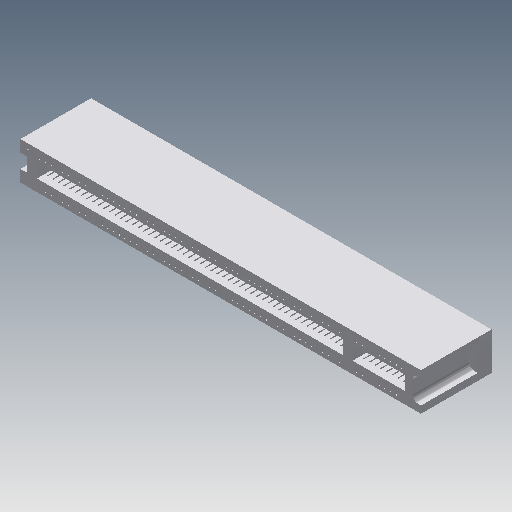
# Autodesk Inventor part: config - pci slot
Saved by Autodesk Inventor 2020 (Build 240152000, 152)
## iProperties
Created: 2005-12-05
Part Number: config - pci slot
Document SubType Name: Modeling
Designer: Simon.Ng@autodesk.com
Stock Number: config - pci slot
Density: 1 g/cm^3
Material: Generic
Mass: 7.81096 g
Surface Area: 89.1874 cm^2
Volume: 7.81096 cm^3
Appearance: Snow
Company: Autodesk Asia Pte. Ltd.
Title: PC Demo
Author: Simon.Ng@autodesk.com
Autodesk Inventor part; units mm, degrees
ref_plane "YZ Plane" through (0, 0, 0) normal (1, 0, 0) x (0, 1, 0)
ref_plane "XZ Plane" through (0, 0, 0) normal (0, 1, 0) x (-1, 0, 0)
ref_plane "XY Plane" through (0, 0, 0) normal (0, 0, 1) x (1, 0, 0)
sketch "Sketch1" plane through (0, 0, 0) normal (0, 0, 1) x (1, 0, 0)
  line L0 (0, 6.4) -> (0, -4.8) construction
  line L1 (-51, 0) -> (68, 0) construction
  line L2 (-42.5, 4) -> (42.5, 4)
  line L3 (42.5, 4) -> (42.5, -4)
  line L4 (42.5, -4) -> (-42.5, -4)
  line L5 (-42.5, -4) -> (-42.5, 4)
  dimension "d0" = 85
  dimension "d1" = 8
  constraints: 8 end point, 2 parallel, 1 horizontal, 1 perpendicular, 2 other
  measures "d0" distance of L2.start L2.end
  measures "d1" distance of L4.end L2.start
extrude "Extrusion1" add sketch "Sketch1" along normal blind 15
sketch "Sketch2" plane through (0, 0, 15) normal (0, 0, 1) x (1, 0, 0)
  line L0 (42.5, 4) -> (42.5, -4) projected
  line L1 (-42.5, -4) -> (-42.5, 4) projected
  line L2 (-42.5, 0) -> (42.5, 0) construction
  line L3 (-42.5, 1.5) -> (-41, 1.5)
  line L4 (-41, 1.5) -> (-41, -1.5)
  line L5 (-41, -1.5) -> (-42.5, -1.5)
  line L6 (-42.5, -1.5) -> (-42.5, 1.5)
  line L7 (42.5, 2.5) -> (41.9, 2.5)
  line L8 (40.7, 1.3) -> (40.7, -1.3)
  line L9 (41.9, -2.5) -> (42.5, -2.5)
  line L10 (42.5, -2.5) -> (42.5, 2.5)
  arc A0 (41.9, 2.5) -> (40.7, 1.3) centre (41.9, 1.3) ccw
  arc A1 (40.7, -1.3) -> (41.9, -2.5) centre (41.9, -1.3) ccw
  point P0 (40.7, -2.5)
  point P1 (40.7, 2.5)
  dimension "d4" = 3
  dimension "d5" = 1.5
  dimension "d6" = 1.8
  dimension "d7" = 5
  dimension "d8" = 1.2
  constraints: 18 end point, 6 point on line, 4 parallel, 4 point on circle, 4 tangent, 2 centre point, 2 horizontal, 2 midpoint, 2 perpendicular, 1 equal radius, 2 other
  measures "d4" distance of L3.end L4.end
  measures "d5" distance of L3.start L3.end
  measures "d6" distance of L7.start point (40.7, 2.5)
  measures "d7" distance of point (40.7, 2.5) point (40.7, -2.5)
  measures "d8" radius of A0
extrude "Extrusion2" cut sketch "Sketch2" against normal blind 12
sketch "Sketch3" plane through (0, 0, 15) normal (0, 0, 1) x (1, 0, 0)
  line L0 (40.7, -1.3) -> (40.7, 1.3) projected
  line L1 (-42.5, 4) -> (42.5, 4) projected
  line L2 (-42.5, 1.5) -> (-42.5, 4) projected
  line L3 (-42.5, 1.5) -> (-41, 1.5) projected
  line L4 (-41, 1.5) -> (-41, -1.5) projected
  line L5 (-41, 0) -> (40.7, 0) construction
  line L6 (-39, 1.5) -> (26, 1.5)
  line L7 (26, 1.5) -> (26, -1.5)
  line L8 (26, -1.5) -> (-39, -1.5)
  line L9 (-39, -1.5) -> (-39, 1.5)
  line L10 (28, 1.5) -> (39.2, 1.5)
  line L11 (39.2, 1.5) -> (39.2, -1.5)
  line L12 (39.2, -1.5) -> (28, -1.5)
  line L13 (28, -1.5) -> (28, 1.5)
  line L14 (-40.634, 3) -> (-41.933, 2.25)
  line L15 (-41.933, 2.25) -> (-41.933, 3.75)
  line L16 (-41.933, 3.75) -> (-40.634, 3)
  point P0 (-41.5, 3)
  dimension "d11" = 2
  dimension "d12" = 2
  dimension "d13" = 65
  dimension "d14" = 1.5
  dimension "d15" = 1
  dimension "d16" = 1
  dimension "d17" = 1.5
  constraints: 24 end point, 5 parallel, 2 horizontal, 2 midpoint, 2 perpendicular, 1 collinear, 1 vertical, 7 other
  measures "d11" distance between parallel lines of L13 L7
  measures "d12" distance between parallel lines of L4 L9
  measures "d13" distance of L6.start L6.end
  measures "d14" distance between parallel lines of L0 L11
  measures "d15" distance from line of L2 point (-41.5, 3)
  measures "d16" distance from line of point (-41.5, 3) L1
  measures "d17" distance of L14.end L15.end
extrude "Extrusion3" cut sketch "Sketch3" against normal blind 8 contours L6 L7 L8 L9 | L10 L11 L12 L13
extrude "Extrusion4" cut sketch "Sketch3" against normal blind 0.1 contours L14 L15 L16
sketch "Sketch4" plane through (0, 0, 15) normal (0, 0, 1) x (1, 0, 0)
  line L0 (-42.5, 1.5) -> (-42.5, 4) projected
  line L1 (-41, 1.5) -> (-41, -1.5) projected
  line L2 (-42.5, 2.75) -> (-33.1148, 2.75) construction
  line L3 (-38.5, 3.25) -> (-38.25, 3.25)
  line L4 (-38.25, 3.25) -> (-38.25, 2.25)
  line L5 (-38.25, 2.25) -> (-38.5, 2.25)
  line L6 (-38.5, 2.25) -> (-38.5, 3.25)
  line L7 (-41, 0) -> (-34.9594, 0) construction
  line L8 (-38.5, -3.25) -> (-38.25, -3.25)
  line L9 (-38.25, -3.25) -> (-38.25, -2.25)
  line L10 (-38.25, -2.25) -> (-38.5, -2.25)
  line L11 (-38.5, -2.25) -> (-38.5, -3.25)
  dimension "d22" = 0.25
  dimension "d23" = 1
  dimension "d24" = 4
  constraints: 20 end point, 4 symmetric about line, 3 perpendicular, 2 midpoint, 2 parallel, 1 horizontal, 1 other
  measures "d22" distance of L3.start L3.end
  measures "d23" distance of L3.end L4.end
  measures "d24" distance between parallel lines of L0 L6
extrude "Extrusion5" cut sketch "Sketch4" against normal blind 8
sketch "Sketch5" plane through (-38.5, 3.25, 7) normal (0, -1, 0) x (1, 0, 0)
  line L0 (0.25, 0) -> (0, 0) projected
  line L1 (0.25, 8) -> (0.25, 0) projected
  line L2 (0, 8) -> (0.25, 8) projected
  line L3 (0, 8) -> (0, 0) projected
  line L4 (0, 6.5) -> (0.25, 6.5)
  dimension "d27" = 1.5
  constraints: 2 end point, 2 point on line, 1 perpendicular
  measures "d27" distance between parallel lines of L4 L2
extrude "Extrusion6" cut sketch "Sketch5" along normal up to surface (6.5 mm away) contours L0 L3 L4 L1
pattern_linear "Rectangular Pattern1" count 65 spacing 1.2 along (1, 0, 0) of "Extrusion6", "Extrusion5" skipped copies 55 56
equation "\"d15\" = d16"
body "Solid1"
